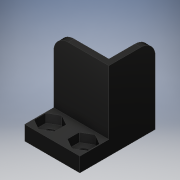
# Autodesk Inventor part: EquerreBatterieDroite
Saved by Autodesk Inventor 2019 (Build 230136000, 136)
## iProperties
Created: 2019-07-30
Part Number: EquerreBatterieDroite
Material: Plastique ABS
Document SubType Name: Modeling
Designer: Sébastien DI MERCURIO
Mass: 14.1383 g
Surface Area: 34.18 cm^2
Volume: 13.338 cm^3
Density: 1.06 g/cm^3
Appearance: Lustré - Noir
Author: Sébastien DI MERCURIO
Autodesk Inventor part; units mm, degrees
ref_plane "YZ Plane" through (0, 0, 0) normal (1, 0, 0) x (0, 1, 0)
ref_plane "XZ Plane" through (0, 0, 0) normal (0, 1, 0) x (-1, 0, 0)
ref_plane "XY Plane" through (0, 0, 0) normal (0, 0, 1) x (1, 0, 0)
sketch "Esquisse1" plane through (0, 0, 0) normal (0, 0, 1) x (1, 0, 0)
  line L0 (0, 0) -> (19, 0)
  line L1 (19, 0) -> (19, 27)
  line L2 (19, 27) -> (0, 27)
  line L3 (0, 27) -> (0, 0)
  dimension "d0" = 27
  dimension "d1" = 19
  constraints: 8 end point, 2 parallel, 1 horizontal, 1 perpendicular
  measures "d0" distance of L0.end L1.end
  measures "d1" distance of L0.start L0.end
extrude "Extrusion1" add sketch "Esquisse1" along normal blind 26
sketch "Esquisse2" plane through (0, 27, 0) normal (0, 1, 0) x (1, 0, 0)
  line L0 (0, 0) -> (0, -14)
  line L1 (0, -14) -> (17, -14)
  line L2 (17, -14) -> (17, 0)
  line L3 (0, 0) -> (0, -26) projected
  line L4 (19, 0) -> (19, -26) projected
  line L5 (0, -26) -> (19, -26)
  line L6 (19, -26) -> (19, -16)
  line L7 (19, -16) -> (0, -16)
  line L8 (0, -16) -> (0, -26)
  line L9 (0, 0) -> (17, 0)
  line L10 (0, 0) -> (19, 0) projected
  dimension "d5" = 2
  dimension "d7" = 10
  dimension "d21" = 2
  dimension "d22" = 14
  constraints: 16 end point, 3 parallel, 1 collinear, 1 horizontal, 1 perpendicular, 1 point on line
  measures "d5" distance between parallel lines of L7 L1
  measures "d7" distance between parallel lines of L5 L7
  measures "d21" distance between parallel lines of L4 L2
  measures "d22" distance between parallel lines of L1 L9
extrude "Extrusion7" cut sketch "Esquisse2" against normal blind 22 contours L9 L2 L1 L0 | L7 L4 L5 L3
sketch "Esquisse5" plane through (0, 5, 0) normal (0, 1, 0) x (1, 0, 0)
  circle A0 centre (3.75, -21) radius 1.5
  circle A1 centre (15.25, -21) radius 1.5
  line L0 (19, -26) -> (0, -26) projected
  line L1 (19, -16) -> (19, -26) projected
  line L2 (0, -26) -> (0, -16) projected
  point P0 (0, 0)
  dimension "d33" = 3
  dimension "d34" = 11.5
  dimension "d35" = 5
  dimension "d36" = 19
  dimension "d37" = 3.75
  constraints: 2 centre point, 1 equal radius, 1 horizontal alignment
  measures "d33" diameter of A0
  measures "d34" distance of A1.centre A0.centre
  measures "d35" distance from line of L0 A0.centre
  measures "d36" distance between parallel lines of L1 L2
  measures "d37" distance from line of A0.centre L2
extrude "Extrusion8" cut sketch "Esquisse5" against normal through all
sketch "Esquisse6" plane through (0, 5, 0) normal (0, 1, 0) x (1, 0, 0)
  circle A0 centre (3.75, -21) radius 1.5 projected
  line L0 (3.75, -16.9585) -> (7.25, -18.9793)
  line L1 (7.25, -18.9793) -> (7.25, -23.0207)
  line L2 (7.25, -23.0207) -> (3.75, -25.0415)
  line L3 (3.75, -25.0415) -> (0.25, -23.0207)
  line L4 (0.25, -23.0207) -> (0.25, -18.9793)
  line L5 (0.25, -18.9793) -> (3.75, -16.9585)
  circle A1 centre (15.25, -21) radius 1.5 projected
  line L6 (15.25, -16.9585) -> (18.75, -18.9793)
  line L7 (18.75, -18.9793) -> (18.75, -23.0207)
  line L8 (18.75, -23.0207) -> (15.25, -25.0415)
  line L9 (15.25, -25.0415) -> (11.75, -23.0207)
  line L10 (11.75, -23.0207) -> (11.75, -18.9793)
  line L11 (11.75, -18.9793) -> (15.25, -16.9585)
  point P0 (0, 0)
  dimension "d40" = 7
  constraints: 24 end point, 2 coincident, 2 vertical alignment, 1 parallel, 26 other
  measures "d40" distance between parallel lines of L1 L4
extrude "Extrusion9" cut sketch "Esquisse6" against normal blind 3
fillet "Congé3" radius 5 2 edges at (0, 27, 15) (18, 27, 0)
equation "\"d21\" = d5"
equation "\"d37\" = -0.5 * d34 + 0.5 * d36"
